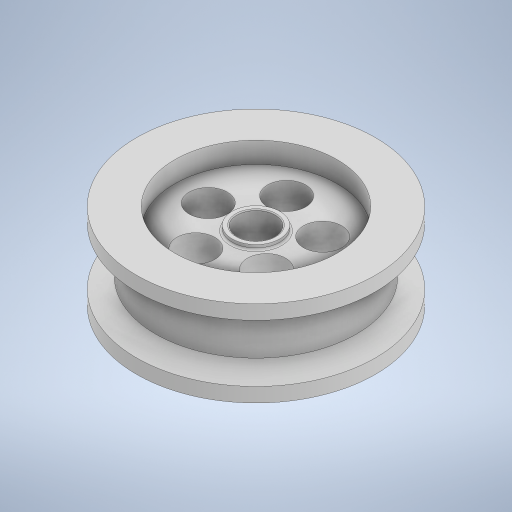
# Autodesk Inventor part: Pulley nhỏ
Saved by Autodesk Inventor 2023 (Build 270158000, 158)
## iProperties
Created: 2023-10-04
Part Number: Pulley nhỏ
Material: Generic
Document SubType Name: Modeling
Designer: huy20
Density: 1 g/cm^3
Appearance: Default
Author: huy20
Autodesk Inventor part; units mm, degrees
ref_plane "YZ Plane" through (0, 0, 0) normal (1, 0, 0) x (0, 1, 0)
ref_plane "XZ Plane" through (0, 0, 0) normal (0, 1, 0) x (-1, 0, 0)
ref_plane "XY Plane" through (0, 0, 0) normal (0, 0, 1) x (1, 0, 0)
sketch "Sketch1" plane through (0, 0, 0) normal (0, 0, 1) x (1, 0, 0)
  line L0 (0, 17.0681) -> (0, -16.825)
  line L1 (2, 2.3018) -> (2, -2.3018)
  line L2 (2, -2.3018) -> (8.5, -2.3018)
  line L3 (8.5, -2.3018) -> (8.5, -4.5)
  line L4 (8.5, -4.5) -> (12.5, -4.5)
  line L5 (12.5, -4.5) -> (12.5, 4.5)
  line L6 (12.5, 4.5) -> (8.5, 4.5)
  line L7 (8.5, 4.5) -> (8.5, 2.3018)
  line L8 (8.5, 2.3018) -> (2, 2.3018)
  line L9 (12.5, 3) -> (10.5, 1.8453)
  line L10 (10.5, 1.8453) -> (10.5, -1.8453)
  line L11 (10.5, -1.8453) -> (12.5, -3)
  point P0 (0, 0)
  point P1 (0, 0.1215)
  point P2 (2, 0)
  dimension "d0" = 25
  dimension "d1" = 4
  dimension "d2" = 4
  dimension "d3" = 9
  dimension "d4" = 1.5
  dimension "d5" = 1.5
  dimension "d6" = 2
  dimension "d7" = 60
  constraints: 24 end point, 6 perpendicular, 4 point on line, 3 vertical, 2 equal length, 2 midpoint, 1 horizontal alignment, 1 other
  measures "d0" diameter of L5 L0
  measures "d1" diameter of L1 L0
  measures "d2" distance of L5.end L6.end
  measures "d3" distance of L4.end L5.end
  measures "d4" distance of L5.end L9.start
  measures "d5" distance of L4.end L11.end
  measures "d6" distance between parallel lines of L5 L10
  measures "d7" angle of L5 L11
revolve "Revolution1" add sketch "Sketch1" angle 360 about axis through (0, 17.0681, 0) along (0, -1, 0) contours L8 L7 L6 L5 L9 L10 L11 L4 L3 L2 L1
sketch "Sketch2" plane through (0, -2.3018, 0) normal (0, -1, 0) x (1, 0, 0)
  circle A0 centre (0, 0) radius 2 construction
  circle A1 centre (0, 0) radius 5 construction
  circle A2 centre (-5, 0) radius 2
  circle A3 centre (-1.5451, -4.7553) radius 2
  circle A4 centre (4.0451, -2.9389) radius 2
  circle A5 centre (4.0451, 2.9389) radius 2
  circle A6 centre (-1.5451, 4.7553) radius 2
  point P0 (0, 0)
  dimension "d9" = 10
  dimension "d10" = 4
  dimension "d13" = 360
  constraints: 5 centre point, 1 coincident, 1 horizontal alignment, 13 other
  measures "d10" diameter of A2
extrude "Extrusion1" cut sketch "Sketch2" against normal through all
sketch "Sketch3" plane through (0, 2.3018, 0) normal (0, 1, 0) x (1, 0, 0)
  circle A0 centre (0, 0) radius 2.5
  circle A1 centre (0, 0) radius 2
  point P0 (0, 0)
  dimension "d17" = 5
  constraints: 2 centre point, 2 coincident
  measures "d17" diameter of A0
extrude "Extrusion2" add sketch "Sketch3" along normal blind 0.5
mirror "Mirror1" about plane through (0, 0, 0) normal (0, 1, 0) of "Extrusion2"
fillet "Fillet1" radius 0.2 1 edges at (-2.5, 2.3018, 0)
fillet "Fillet2" radius 0.2 1 edges at (-2.5, -2.3018, 0)
fillet "Fillet3" radius 0.1 2 edges at (-2, 2.8018, 0) (-2, -2.8018, 0)
body "Solid1"
